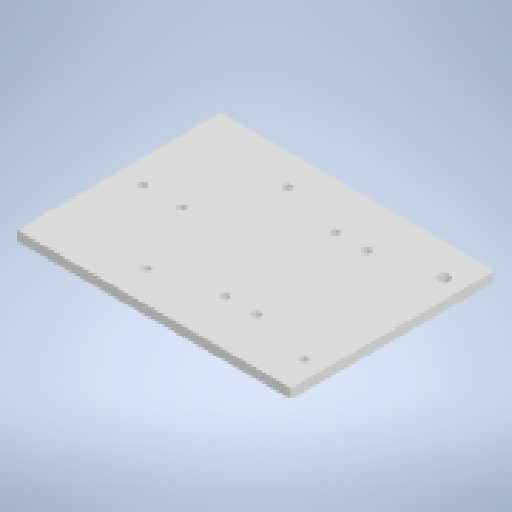
# Autodesk Inventor part: C beam gantry (big side y axis)
Saved by Autodesk Inventor 2023.2 (Build 272271000, 271)
## iProperties
Created: 2023-03-20
Part Number: C beam gantry (big side y axis)
Material: Generic
Document SubType Name: Modeling
Designer: dmargari
Density: 1 g/cm^3
Appearance: Default
Author: dmargari
Autodesk Inventor part; units mm, degrees
ref_plane "YZ Plane" through (0, 0, 0) normal (1, 0, 0) x (0, 1, 0)
ref_plane "XZ Plane" through (0, 0, 0) normal (0, 1, 0) x (-1, 0, 0)
ref_plane "XY Plane" through (0, 0, 0) normal (0, 0, 1) x (1, 0, 0)
sketch "Sketch1" plane through (0, 0, 0) normal (0, 1, 0) x (-1, 0, 0)
  line L0 (185.092, -257.4018) -> (60.092, -257.4018)
  line L1 (60.092, -257.4018) -> (60.092, -387.4018)
  line L2 (60.092, -387.4018) -> (185.092, -387.4018)
  line L3 (185.092, -387.4018) -> (185.092, -257.4018) construction
  line L4 (172.792, -257.4018) -> (172.792, -387.4018) construction
  line L5 (72.392, -257.4018) -> (72.392, -387.4018) construction
  circle A0 centre (172.792, -277.4018) radius 2.55
  circle A1 centre (172.792, -367.4018) radius 2.55
  circle A2 centre (72.392, -277.4018) radius 2.55
  circle A3 centre (72.392, -367.4018) radius 3.55
  line L6 (185.092, -257.4018) -> (235.092, -257.4018)
  line L7 (235.092, -257.4018) -> (235.092, -387.4018)
  line L8 (235.092, -387.4018) -> (185.092, -387.4018)
  point P0 (0, 0)
  point P1 (-73.8984, 140.5937)
  dimension "d0" = 125
  dimension "d1" = 130
  dimension "d2" = 12.3
  dimension "d3" = 12.3
  dimension "d4" = 5.1
  dimension "d5" = 5.1
  dimension "d6" = 5.1
  dimension "d7" = 7.1
  dimension "d8" = 50
  dimension "d23" = 20
  dimension "d24" = 20
  dimension "d25" = 20
  dimension "d26" = 20
  constraints: 18 end point, 9 point on line, 4 centre point, 4 perpendicular, 2 horizontal, 2 parallel, 1 collinear
  measures "d0" distance of L2.end L1.end
  measures "d1" distance of L1.end L0.end
  measures "d2" distance between parallel lines of L1 L5
  measures "d3" distance between parallel lines of L3 L4
  measures "d4" diameter of A0
  measures "d5" diameter of A1
  measures "d6" diameter of A2
  measures "d7" diameter of A3
  measures "d8" distance of L0.start L6.end
  measures "d23" distance from line of L2 A1.centre
  measures "d24" distance from line of L2 A3.centre
  measures "d25" distance from line of L0 A0.centre
  measures "d26" distance from line of L0 A2.centre
extrude "Extrusion1" add sketch "Sketch1" along normal blind 6
fillet "Fillet1" radius 2 2 edges at (-60.092, 3, -257.4018) (-60.092, 3, -387.4018)
sketch "Sketch2" plane through (0, 6, 0) normal (0, 1, 0) x (1, 0, 0)
  line L0 (-235.092, 387.4018) -> (-235.092, 257.4018) construction
  line L1 (-235.092, 322.4018) -> (-60.092, 322.4018) construction
  line L2 (-60.092, 259.4018) -> (-60.092, 385.4018) construction
  line L3 (-235.092, 312.4018) -> (-30.092, 312.4018) construction
  line L4 (-235.092, 332.4018) -> (-30.092, 332.4018) construction
  line L5 (-235.092, 257.4018) -> (-62.092, 257.4018) construction
  line L6 (-220.092, 257.4018) -> (-220.092, 387.4018) construction
  line L7 (-62.092, 387.4018) -> (-235.092, 387.4018) construction
  line L8 (-195.092, 257.4018) -> (-195.092, 387.4018) construction
  point P0 (0, 0)
  point P1 (-220.092, 322.4018)
  point P2 (-195.092, 322.4018)
  dimension "d12" = 10
  dimension "d13" = 10
  dimension "d14" = 15
  dimension "d15" = 25
  constraints: 10 end point, 4 midpoint, 2 parallel, 2 point on line, 2 vertical
  measures "d12" distance between parallel lines of L1 L3
  measures "d13" distance between parallel lines of L1 L4
  measures "d14" distance between parallel lines of L0 L6
  measures "d15" distance between parallel lines of L8 L6
hole "Hole1" at (-220.092, 6, -322.4018) at (-195.092, 6, -322.4018) direction (0, -1, 0) diameter 5.1 end through all
sketch "Sketch3" plane through (0, 6, 0) normal (0, 1, 0) x (1, 0, 0)
  circle A0 centre (-112.092, 287.4018) radius 2.55 projected
  circle A1 centre (-132.092, 287.4018) radius 2.55 projected
  circle A2 centre (-132.092, 357.4018) radius 2.55 projected
  circle A3 centre (-112.092, 357.4018) radius 2.55 projected
  point P0 (0, 0)
hole "Hole2" at (-132.092, 6, -287.4018) at (-112.092, 6, -287.4018) at (-112.092, 6, -357.4018) at (-132.092, 6, -357.4018) direction (0, -1, 0) diameter 5.1 end through all
body "Solid1"
